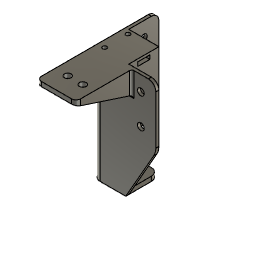
Frame Leg V2 - Rear Left (Autodesk Fusion 360 design; units mm, degrees)
Autodesk Fusion 360 part; units mm, degrees
sketch "Sketch1" plane through (0, 0, 0) normal (0, 0, 1) x (1, 0, 0) in component "Frame Leg"
  line L0 (0, 0) -> (0, 42)
  line L1 (0, 42) -> (2, 42)
  line L2 (2, 42) -> (2, 22)
  line L3 (2, 22) -> (22, 22)
  line L4 (22, 22) -> (22, 2)
  line L5 (0, 0) -> (42, 0)
  line L6 (42, 0) -> (42, 2)
  line L7 (42, 2) -> (22, 2)
  dimension "d1" = 42
  dimension "d2" = 2
  dimension "d3" = 20
  dimension "d4" = 20
  dimension "d5" = 20
  dimension "d6" = 42
  dimension "d7" = 2
  constraint coincident L0.start L5.start
  constraint vertical L0
  constraint perpendicular L0 L1
  constraint perpendicular L1 L2
  constraint perpendicular L2 L3
  constraint perpendicular L3 L4
  constraint perpendicular L0 L5
  constraint perpendicular L5 L6
  measures "d1" distance of L0.start L0.end
  measures "d2" distance of L0.end L1.end
  measures "d3" distance of L1.end L2.end
  measures "d4" distance of L2.end L3.end
  measures "d5" distance of L3.end L4.end
  measures "d6" distance of L0.start L5.end
  measures "d7" distance of L5.end L6.end
extrude "Extrude1" add sketch "Sketch1" along normal blind 75 in component "Frame Leg"
sketch "Sketch2" plane through (22, 0, 0) normal (1, 0, 0) x (0, 1, 0) in component "Frame Leg"
  line L0 (2, 0) -> (22, 0)
  line L1 (22, 0) -> (22, 75)
  line L2 (22, 75) -> (2, 75)
  line L3 (2, 75) -> (2, 0)
  line L4 (2, 0) -> (2, 75)
  line L5 (2, 75) -> (22, 75)
  line L6 (22, 0) -> (22, 75)
  line L7 (22, 0) -> (2, 0)
  line L8 (2, 35) -> (22, 35)
  line L9 (2, 3) -> (22, 3)
  line L10 (2, 35) -> (2, 3)
  line L11 (22, 35) -> (22, 3)
  dimension "d10" = 40
  dimension "d11" = 3
  constraint coincident L4 L8.start
  constraint coincident L6 L8.end
  constraint perpendicular L6 L8
  constraint coincident L4 L9.start
  constraint coincident L6 L9.end
  constraint perpendicular L6 L9
  measures "d10" distance of L2 L8
  measures "d11" distance of L7 L9
extrude "Extrude2" cut sketch "Sketch2" against normal up to surface (20 mm away) contours L1 L3 L4 L6 L8 L9 L10 L11 in component "Frame Leg"
sketch "Sketch16" plane through (0, 0, 0) normal (0, 0, -1) x (1, 0, 0) in component "Frame Leg"
  line L0 (42, 0) -> (0, 0)
  line L1 (0, 0) -> (0, -42)
  line L2 (0, -42) -> (2, -42)
  line L3 (2, -42) -> (2, -22)
  line L4 (2, -22) -> (22, -22)
  line L5 (22, -22) -> (22, -2)
  line L6 (22, -2) -> (42, -2)
  line L7 (42, -2) -> (42, 0)
  line L8 (12, -22) -> (12, 0) construction
  line L9 (22, -12) -> (0, -12) construction
  circle A0 centre (12, -12) radius 2.6
  dimension "d145" = 5.2
  constraint midpoint L4 L8.start
  constraint coincident L0 L8.end
  constraint perpendicular L0 L8
  constraint midpoint L5 L9.start
  constraint coincident L1 L9.end
  constraint perpendicular L1 L9
  constraint coincident L8 A0.centre
  constraint coincident L9 A0.centre
  measures "d145" diameter of A0
extrude "Extrude17" cut sketch "Sketch16" against normal blind 3 contours A0 in component "Frame Leg"
sketch "Sketch3" plane through (0, 2, 0) normal (0, 1, 0) x (-1, 0, 0) in component "Frame Leg"
  line L0 (-42, 0) -> (-22, 0)
  line L1 (-22, 0) -> (-22, 3)
  line L2 (-22, 3) -> (-2, 3)
  line L3 (-2, 3) -> (-2, 35)
  line L4 (-2, 35) -> (-22, 35)
  line L5 (-22, 35) -> (-22, 75)
  line L6 (-22, 75) -> (-42, 75)
  line L7 (-42, 75) -> (-42, 0)
  line L8 (-42, 0) -> (-42, 75)
  line L9 (-42, 75) -> (-22, 75)
  line L10 (-22, 35) -> (-22, 75)
  line L11 (-22, 35) -> (-2, 35)
  line L12 (-2, 3) -> (-2, 35)
  line L13 (-22, 3) -> (-2, 3)
  line L14 (-22, 0) -> (-22, 3)
  line L15 (-42, 0) -> (-22, 0)
  line L16 (-42, 35) -> (-42, 0)
  line L17 (-22, 0) -> (-42, 0)
  line L18 (-2, 35) -> (-42, 35) construction
  line L19 (-22, 0) -> (-42, 35)
  dimension "d53" = 40
  constraint coincident L8 L16.start
  constraint coincident L0.start L7.end
  constraint coincident L0.end L1.start
  constraint coincident L3 L4.start
  constraint perpendicular L3 L18
  measures "d53" distance of L9 L18
extrude "Extrude3" cut sketch "Sketch3" against normal blind 2 contours L0 L7 L8 L15 L16 L17 L19 in component "Frame Leg"
sketch "Sketch4" plane through (2, 0, 0) normal (1, 0, 0) x (0, 1, 0) in component "Frame Leg"
  line L0 (22, 0) -> (42, 0)
  line L1 (42, 0) -> (42, 75)
  line L2 (42, 75) -> (22, 75)
  line L3 (22, 75) -> (22, 35)
  line L4 (22, 35) -> (2, 35)
  line L5 (2, 35) -> (2, 3)
  line L6 (2, 3) -> (22, 3)
  line L7 (22, 3) -> (22, 0)
  line L8 (2, 3) -> (2, 35)
  line L9 (2, 35) -> (22, 35)
  line L10 (22, 3) -> (2, 3)
  line L11 (22, 0) -> (22, 3)
  line L12 (42, 0) -> (22, 0)
  line L13 (42, 0) -> (42, 75)
  line L14 (22, 75) -> (42, 75)
  line L15 (22, 35) -> (22, 75)
  line L16 (22, 0) -> (42, 0)
  line L17 (42, 0) -> (42, 35)
  line L18 (2, 35) -> (42, 35) construction
  line L19 (42, 35) -> (22, 0)
  dimension "d56" = 40
  constraint coincident L13 L17.end
  constraint coincident L0.start L7.end
  constraint coincident L0.end L1.start
  constraint horizontal L18
  constraint coincident L5 L4.end
  constraint coincident L17 L18.end
  measures "d56" distance of L14 L18
extrude "Extrude4" cut sketch "Sketch4" against normal up to surface (2 mm away) contours L0 L1 L12 L13 L16 L17 L19 in component "Frame Leg"
fillet "Fillet1" radius 10 1 edges at (42, 1, 35) in component "Frame Leg"
fillet "Fillet1" radius 10 1 edges at (1, 42, 35) in component "Frame Leg"
fillet "Fillet4" radius 5 2 edges at (42, 1, 75) (1, 42, 75) in component "Frame Leg"
sketch "Sketch5" plane through (0, 0, 0) normal (-1, 0, 0) x (0, -1, 0) in component "Frame Leg"
  line L0 (-22, 0) -> (0, 0)
  line L1 (0, 75) -> (-37, 75)
  line L2 (-22, 35) -> (-22, 75)
  line L3 (-42, 37.6556) -> (-42, 70)
  line L4 (-22, 75) -> (-37, 75)
  line L5 (-42, 65) -> (-22, 65) construction
  line L6 (-42, 45) -> (-22, 45) construction
  line L7 (-32, 75) -> (-32, 45) construction
  circle A0 centre (-32, 65) radius 2.25
  circle A1 centre (-32, 45) radius 2.25
  line L8 (-42, 70) -> (-42, 37.6556)
  line L9 (-40.6824, 32.6943) -> (-22, 0)
  arc A2 (-42, 37.6556) -> (-40.6824, 32.6943) centre (-32, 37.6556) ccw
  arc A3 (-37, 75) -> (-42, 70) centre (-37, 70) ccw
  line L10 (0, 0) -> (0, 75)
  dimension "d28" = 10
  dimension "d29" = 30
  dimension "d30" = 10
  dimension "d32" = 4.5
  dimension "d34" = 4.5
  constraint coincident L3 L5.start
  constraint coincident L2 L5.end
  constraint perpendicular L2 L5
  constraint coincident L3 L6.start
  constraint coincident L2 L6.end
  constraint perpendicular L2 L6
  constraint coincident L1 L7.start
  constraint coincident L6 L7.end
  constraint perpendicular L6 L7
  constraint coincident L7 A0.centre
  constraint coincident L5 A0.centre
  constraint coincident L7.end A1.centre
  measures "d28" distance of L4 L5
  measures "d29" distance of L4 L6
  measures "d30" distance of L3 L7
  measures "d32" diameter of A0
  measures "d34" diameter of A1
extrude "Extrude5" cut sketch "Sketch5" against normal blind 2 contours A0 | A1 in component "Frame Leg"
sketch "Sketch7" plane through (0, 0, 0) normal (-1, 0, 0) x (0, -1, 0) in component "Frame Leg"
  circle A0 centre (-32, 65) radius 2.25
  circle A1 centre (-32, 45) radius 2.25
  arc A2 (-37, 75) -> (-42, 70) centre (-37, 70) ccw
  line L0 (-42, 70) -> (-42, 37.6556)
  arc A3 (-42, 37.6556) -> (-40.6824, 32.6943) centre (-32, 37.6556) ccw
  line L1 (-40.6824, 32.6943) -> (-22, 0)
  line L2 (-22, 0) -> (0, 0)
  line L3 (0, 75) -> (-37, 75)
  line L4 (-2, 35) -> (-2, 75)
  line L5 (-2, 75) -> (-22, 75)
  line L6 (-22, 35) -> (-22, 75)
  line L7 (-22, 45) -> (-2, 45) construction
  line L8 (-2, 35) -> (-22, 35)
  line L9 (-12, 75) -> (-12, 35) construction
  circle A4 centre (-12, 45) radius 2.75
  line L10 (0, 0) -> (0, 75)
  dimension "d68" = 30
  dimension "d70" = 10
  dimension "d72" = 5.5
  constraint coincident L6 L7.start
  constraint coincident L4 L7.end
  constraint perpendicular L4 L7
  constraint coincident L5 L9.start
  constraint coincident L8 L9.end
  constraint perpendicular L8 L9
  constraint midpoint L7 A4.centre
  measures "d68" distance of L5 L7
  measures "d70" distance of L4 L9
  measures "d72" diameter of A4
extrude "Extrude7" cut sketch "Sketch7" against normal blind 22 contours A4 in component "Frame Leg"
sketch "Sketch8" plane through (0, 0, 0) normal (-1, 0, 0) x (0, -1, 0) in component "Frame Leg"
  circle A0 centre (-12, 45) radius 2.75
  circle A1 centre (-32, 65) radius 2.25
  circle A2 centre (-32, 45) radius 2.25
  arc A3 (-37, 75) -> (-42, 70) centre (-37, 70) ccw
  line L0 (-42, 70) -> (-42, 37.6556)
  arc A4 (-42, 37.6556) -> (-40.6824, 32.6943) centre (-32, 37.6556) ccw
  line L1 (-40.6824, 32.6943) -> (-22, 0)
  line L2 (-22, 0) -> (0, 0)
  line L3 (0, 75) -> (-37, 75)
  circle A5 centre (-12, 45) radius 5
  line L4 (0, 0) -> (0, 75)
  dimension "d76" = 10
  constraint concentric A0 A5
  measures "d76" diameter of A5
extrude "Extrude8" cut sketch "Sketch8" against normal blind 17 contours A5 in component "Frame Leg"
sketch "Sketch6" plane through (0, 0, 0) normal (0, -1, 0) x (1, 0, 0) in component "Frame Leg"
  line L0 (42, 37.6556) -> (42, 70)
  line L1 (37, 75) -> (0, 75)
  line L2 (0, 0) -> (22, 0)
  line L3 (22, 35) -> (22, 75)
  line L4 (42, 37.6556) -> (42, 70)
  line L5 (37, 75) -> (22, 75)
  line L6 (22, 65) -> (42, 65) construction
  line L7 (22, 45) -> (42, 45) construction
  line L8 (12, 75) -> (12, 45) construction
  line L9 (32, 75) -> (32, 45) construction
  circle A0 centre (32, 65) radius 2.25
  circle A1 centre (32, 45) radius 2.25
  line L10 (22, 0) -> (40.6824, 32.6943)
  arc A2 (40.6824, 32.6943) -> (42, 37.6556) centre (32, 37.6556) ccw
  arc A3 (42, 70) -> (37, 75) centre (37, 70) ccw
  line L11 (2, 35) -> (2, 75)
  line L12 (0, 75) -> (0, 0)
  dimension "d38" = 10
  dimension "d39" = 30
  dimension "d40" = 10
  dimension "d43" = 4.5
  dimension "d51" = 4.5
  dimension "d66" = 10
  constraint coincident L3 L6.start
  constraint coincident L4 L6.end
  constraint perpendicular L4 L6
  constraint coincident L3 L7.start
  constraint coincident L4 L7.end
  constraint perpendicular L4 L7
  constraint coincident L1 L8.start
  constraint coincident L7 L8.end
  constraint perpendicular L7 L8
  constraint coincident L5 L9.start
  constraint coincident L7 L9.end
  constraint perpendicular L7 L9
  constraint coincident L9 A0.centre
  constraint coincident L6 A0.centre
  constraint coincident L9.end A1.centre
  measures "d38" distance of L1 L6
  measures "d39" distance of L5 L7
  measures "d40" distance of L4 L9
  measures "d43" diameter of A0
  measures "d51" diameter of A1
  measures "d66" distance of L8 L11
extrude "Extrude6" cut sketch "Sketch6" against normal blind 2 contours A0 | A1 in component "Frame Leg"
sketch "Sketch9" plane through (0, 0, 0) normal (0, -1, 0) x (1, 0, 0) in component "Frame Leg"
  circle A0 centre (32, 65) radius 2.25
  circle A1 centre (32, 45) radius 2.25
  arc A2 (42, 70) -> (37, 75) centre (37, 70) ccw
  line L0 (37, 75) -> (0, 75)
  line L1 (0, 0) -> (22, 0)
  line L2 (22, 0) -> (40.6824, 32.6943)
  arc A3 (40.6824, 32.6943) -> (42, 37.6556) centre (32, 37.6556) ccw
  line L3 (42, 37.6556) -> (42, 70)
  line L4 (2, 35) -> (2, 75)
  line L5 (22, 35) -> (22, 75)
  line L6 (22, 35) -> (2, 35)
  line L7 (22, 75) -> (2, 75)
  line L8 (12, 75) -> (12, 35) construction
  line L9 (2, 65) -> (22, 65) construction
  circle A4 centre (12, 65) radius 2.75
  line L10 (0, 75) -> (0, 0)
  dimension "d79" = 10
  dimension "d80" = 10
  dimension "d82" = 5.5
  constraint coincident L7 L8.start
  constraint coincident L6 L8.end
  constraint perpendicular L6 L8
  constraint coincident L4 L9.start
  constraint coincident L5 L9.end
  constraint perpendicular L5 L9
  constraint midpoint L9 A4.centre
  measures "d79" distance of L4 L8
  measures "d80" distance of L7 L9
  measures "d82" diameter of A4
extrude "Extrude9" cut sketch "Sketch9" against normal up to surface (22 mm away) contours A4 in component "Frame Leg"
sketch "Sketch10" plane through (0, 0, 0) normal (0, -1, 0) x (1, 0, 0) in component "Frame Leg"
  circle A0 centre (12, 65) radius 2.75
  circle A1 centre (32, 65) radius 2.25
  circle A2 centre (32, 45) radius 2.25
  arc A3 (42, 70) -> (37, 75) centre (37, 70) ccw
  line L0 (37, 75) -> (0, 75)
  line L1 (0, 0) -> (22, 0)
  line L2 (22, 0) -> (40.6824, 32.6943)
  arc A4 (40.6824, 32.6943) -> (42, 37.6556) centre (32, 37.6556) ccw
  line L3 (42, 37.6556) -> (42, 70)
  circle A5 centre (12, 65) radius 5
  line L4 (0, 75) -> (0, 0)
  dimension "d86" = 10
  constraint concentric A0 A5
  measures "d86" diameter of A5
extrude "Extrude10" cut sketch "Sketch10" against normal blind 17 contours A5 in component "Frame Leg"
fillet "Fillet9" radius 5 1 edges at (22, 22, 1.5) in component "Frame Leg"
fillet "Fillet10" radius 5 1 edges at (2, 2, 19) in component "Frame Leg"
sketch "Sketch11" plane through (22, 0, 0) normal (1, 0, 0) x (0, 1, 0) in component "Frame Leg"
  circle A0 centre (12, 45) radius 2.75
  line L0 (2, 35) -> (22, 35)
  line L1 (22, 35) -> (22, 75)
  line L2 (22, 75) -> (2, 75)
  line L3 (2, 75) -> (2, 35)
  line L4 (12, 75) -> (12, 35) construction
  line L5 (2, 72) -> (22, 72) construction
  line L6 (16, 73.3) -> (8, 73.3)
  line L7 (8, 73.3) -> (8, 70.7)
  line L8 (8, 70.7) -> (16, 70.7)
  line L9 (16, 70.7) -> (16, 73.3)
  line L10 (16, 73.3) -> (8, 70.7) construction
  line L11 (8, 73.3) -> (16, 70.7) construction
  point P0 (12, 72)
  dimension "d94" = 3
  dimension "d95" = 8
  dimension "d96" = 2.6
  constraint midpoint L2 L4.start
  constraint midpoint L0 L4.end
  constraint coincident L3 L5.start
  constraint coincident L1 L5.end
  constraint perpendicular L1 L5
  constraint horizontal L6
  constraint perpendicular L6 L7
  constraint parallel L6 L8
  constraint parallel L7 L9
  constraint coincident L10 P0
  constraint coincident L11 P0
  constraint midpoint L5 P0
  measures "d94" distance of L2 L5
  measures "d95" distance of L7.end L8.end
  measures "d96" distance of L6.end L7.end
extrude "Extrude11" cut sketch "Sketch11" against normal up to surface (22 mm away) contours L6 L7 L8 L9 in component "Frame Leg"
sketch "Sketch12" plane through (0, 0, 0) normal (0, -1, 0) x (1, 0, 0) in component "Frame Leg"
  circle A0 centre (12, 65) radius 5
  circle A1 centre (32, 65) radius 2.25
  circle A2 centre (32, 45) radius 2.25
  arc A3 (42, 70) -> (37, 75) centre (37, 70) ccw
  line L0 (37, 75) -> (0, 75)
  line L1 (0, 0) -> (22, 0)
  line L2 (22, 0) -> (40.6824, 32.6943)
  arc A4 (40.6824, 32.6943) -> (42, 37.6556) centre (32, 37.6556) ccw
  line L3 (42, 37.6556) -> (42, 70)
  line L4 (0, 75) -> (26, 75)
  line L5 (26, 75) -> (26, 72)
  line L6 (26, 72) -> (0, 72)
  line L7 (0, 72) -> (0, 75)
  line L8 (20, 75) -> (20, 35) construction
  line L9 (13, 72) -> (12, 72) construction
  line L10 (13, 72) -> (14, 72) construction
  line L11 (0, 60) -> (42, 60) construction
  line L12 (0, 75) -> (0, 0)
  line L13 (0, 72) -> (2, 72)
  line L14 (2, 72) -> (2, 60)
  line L15 (2, 60) -> (0, 60)
  line L16 (0, 60) -> (0, 72)
  line L17 (26, 72) -> (24, 72)
  line L18 (24, 72) -> (24, 60)
  line L19 (24, 60) -> (26, 60)
  line L20 (26, 60) -> (26, 72)
  dimension "d99" = 26
  dimension "d100" = 3
  dimension "d101" = 1
  dimension "d102" = 1
  dimension "d103" = 15
  dimension "d134" = 2
  dimension "d135" = 2
  constraint horizontal L4
  constraint vertical L5
  constraint horizontal L6
  constraint vertical L7
  constraint coincident L0.end L4.start
  constraint perpendicular L4 L8
  constraint midpoint L6 L9.start
  constraint perpendicular L8 L9
  constraint perpendicular L8 L10
  constraint coincident L3 L11.end
  constraint perpendicular L3 L11
  constraint coincident L11.start L12
  constraint horizontal L13
  constraint vertical L14
  constraint horizontal L15
  constraint vertical L16
  constraint horizontal L17
  constraint vertical L18
  constraint horizontal L19
  constraint vertical L20
  measures "d99" distance of L0.end L4.end
  measures "d100" distance of L0.end L6.end
  measures "d101" distance of L9.start L9.end
  measures "d102" distance of L9.start L10.end
  measures "d103" distance of L0 L11
  measures "d134" distance of L6.end L13.end
  measures "d135" distance of L5.end L17.end
extrude "Extrude12" add sketch "Sketch12" along normal blind 37 contours L0 L4 L5 L6 L7 L12 L13 L17 | L6 L17 L18 L19 L20 | L6 L12 L13 L14 L15 L16 in component "Frame Leg"
sketch "Sketch13" plane through (26, 0, 0) normal (1, 0, 0) x (0, 1, 0) in component "Frame Leg"
  line L0 (0, 68) -> (0, 72)
  line L1 (-28, 60) -> (0, 60)
  line L2 (0, 60) -> (-37, 72)
  line L3 (0, 60) -> (0, 75)
  line L4 (0, 75) -> (-37, 75)
  line L5 (-37, 75) -> (-37, 60)
  line L6 (-37, 60) -> (0, 60)
  line L7 (0, 72) -> (-37, 72)
  constraint coincident L1.end L2.start
  constraint coincident L2.end L5
  constraint coincident L2.end L7
extrude "Extrude13" cut sketch "Sketch13" against normal up to surface (26 mm away) contours L1 L2 L5 L6 in component "Frame Leg"
fillet "Fillet12" radius 3 2 edges at (26, -37, 73.5) (0, -37, 73.5) in component "Frame Leg"
sketch "Sketch14" plane through (0, 0, 75) normal (0, 0, 1) x (-1, 0, 0) in component "Frame Leg"
  arc A0 (0, 34) -> (-3, 37) centre (-3, 34) ccw
  line L0 (-3, 37) -> (-23, 37)
  arc A1 (-23, 37) -> (-26, 34) centre (-23, 34) ccw
  line L1 (-26, 34) -> (-26, 0)
  line L2 (-26, 0) -> (-37, 0)
  line L3 (-37, 0) -> (-37, -2)
  line L4 (-37, -2) -> (-22, -2)
  line L5 (-22, -2) -> (-22, -22)
  line L6 (-22, -22) -> (-2, -22)
  line L7 (-2, -22) -> (-2, -37)
  line L8 (-2, -37) -> (0, -37)
  line L9 (0, -37) -> (0, 34)
  line L10 (0, 25) -> (-26, 25) construction
  line L11 (-13.5, 37) -> (-13.5, 9) construction
  line L12 (-8.5, 37) -> (-8.5, 9) construction
  line L13 (-18.5, 37) -> (-18.5, 9) construction
  circle A2 centre (-8.5, 25) radius 2.25
  circle A3 centre (-18.5, 25) radius 2.25
  dimension "d115" = 5
  dimension "d116" = 5
  dimension "d117" = 4.5
  dimension "d118" = 4.5
  dimension "d133" = 13.5
  dimension "d136" = 12
  constraint coincident L1 L10.end
  constraint perpendicular L1 L10
  constraint perpendicular L0 L11
  constraint coincident L0 L12.start
  constraint coincident L0 L13.start
  constraint perpendicular L0 L13
  constraint coincident L12 A2.centre
  constraint coincident L10 A2.centre
  constraint coincident L10 A3.centre
  constraint coincident L13 A3.centre
  measures "d115" distance of L11 L12
  measures "d116" distance of L11 L13
  measures "d117" diameter of A2
  measures "d118" diameter of A3
  measures "d133" distance of L9 L11
  measures "d136" distance of L0 L10
extrude "Extrude14" cut sketch "Sketch14" against normal up to surface (3 mm away) contours A2 | A3 in component "Frame Leg"
fillet "Fillet13" radius 1.5 1 edges at (26, 0, 67.5) in component "Frame Leg"
fillet "Fillet14" radius 1.5 1 edges at (13, 0, 72) in component "Frame Leg"
fillet "Fillet14" radius 1.5 1 edges at (25.75, 0, 60) in component "Frame Leg"
sketch "Sketch15" plane through (0, 0, 75) normal (0, 0, 1) x (-1, 0, 0) in component "Frame Leg"
  circle A0 centre (-8.5, 25) radius 2.25
  circle A1 centre (-18.5, 25) radius 2.25
  arc A2 (0, 34) -> (-3, 37) centre (-3, 34) ccw
  line L0 (-3, 37) -> (-23, 37)
  arc A3 (-23, 37) -> (-26, 34) centre (-23, 34) ccw
  line L1 (-26, 34) -> (-26, 1.5)
  arc A4 (-27.5, 0) -> (-26, 1.5) centre (-27.5, 1.5) ccw
  line L2 (-27.5, 0) -> (-37, 0)
  line L3 (-37, 0) -> (-37, -2)
  line L4 (-37, -2) -> (-22, -2)
  line L5 (-22, -2) -> (-22, -22)
  line L6 (-22, -22) -> (-2, -22)
  line L7 (-2, -22) -> (-2, -37)
  line L8 (-2, -37) -> (0, -37)
  line L9 (0, -37) -> (0, 34)
  line L10 (0, -19) -> (-22, -19) construction
  line L11 (0, -3.5) -> (-22, -3.5) construction
  line L12 (-4.5, -22) -> (-4.5, -2) construction
  line L13 (-22, -2) -> (-7, -2) construction
  circle A5 centre (-4.5, -19) radius 1.4
  circle A6 centre (-4.5, -3.5) radius 1.4
  dimension "d125" = 2.5
  dimension "d126" = 3
  dimension "d128" = 2.8
  dimension "d129" = 2.8
  dimension "d132" = 15.5
  constraint coincident L9 L10.start
  constraint coincident L5 L10.end
  constraint perpendicular L5 L10
  constraint coincident L9 L11.start
  constraint coincident L5 L11.end
  constraint perpendicular L5 L11
  constraint coincident L6 L12.start
  constraint perpendicular L11 L12
  constraint coincident L12 A5.centre
  constraint coincident L10 A5.centre
  constraint coincident L12 A6.centre
  constraint coincident L11 A6.centre
  measures "d125" distance of L7 L12
  measures "d126" distance of L6 L10
  measures "d128" diameter of A5
  measures "d129" diameter of A6
  measures "d132" distance of L10 L11
extrude "Extrude15" cut sketch "Sketch15" against normal blind 10 contours A5 | A6 in component "Frame Leg"
fillet "Fillet15" radius 5 1 edges at (0, 0, 30) in component "Frame Leg"
component "Frame Leg" placed x (1, 0, 0) y (0, 1, 0) z (0, 0, 1) at (0, 0, 0)
named bodies: "Frame Leg - Rear Left"
